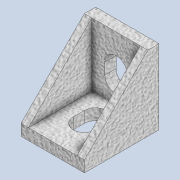
# Autodesk Inventor part: 2020 Extrusion 90deg 2Hole Aluminum Bracket
Saved by Autodesk Inventor 2022 (Build 260153000, 153)
## iProperties
Created: 2021-11-27
Part Number: 2020 Extrusion 90deg 2Hole Aluminum Bracket
Material: Generic
Document SubType Name: Modeling
Designer: Coy
Density: 1 g/cm^3
Appearance: Aluminum Cast
Author: Coy
Autodesk Inventor part; units mm, degrees
ref_plane "YZ Plane" through (0, 0, 0) normal (1, 0, 0) x (0, 1, 0)
ref_plane "XZ Plane" through (0, 0, 0) normal (0, 1, 0) x (-1, 0, 0)
ref_plane "XY Plane" through (0, 0, 0) normal (0, 0, 1) x (1, 0, 0)
sketch "Sketch1" plane through (0, 0, 0) normal (1, 0, 0) x (0, 1, 0)
  line L0 (0, 0) -> (0, 20)
  line L1 (0, 20) -> (3, 20)
  line L2 (3, 20) -> (20, 3)
  line L3 (20, 3) -> (20, 0)
  line L4 (20, 0) -> (0, 0)
  dimension "d0" = 20
  dimension "d1" = 3
  dimension "d2" = 20
  dimension "d3" = 3
  constraints: 10 end point, 2 perpendicular, 1 parallel, 1 vertical
  measures "d0" distance of L0.start L0.end
  measures "d1" distance of L0.end L1.end
  measures "d2" distance of L3.end L0.start
  measures "d3" distance of L2.end L3.end
extrude "Extrusion1" add sketch "Sketch1" along normal blind 2
sketch "Sketch2" plane through (2, 0, 0) normal (1, 0, 0) x (0, 0, -1)
  line L0 (0, 20) -> (-3, 20) projected
  line L1 (-3, 20) -> (-20, 3) projected
  line L2 (-20, 3) -> (-20, 0) projected
  line L3 (-20, 0) -> (0, 0) projected
  line L4 (0, 0) -> (0, 20) projected
  line L5 (-3, 20) -> (-20, 3) projected
  line L6 (-20, 3) -> (-3, 3)
  line L7 (-3, 3) -> (-3, 20)
  constraints: 4 end point, 1 horizontal, 1 perpendicular
extrude "Extrusion2" add sketch "Sketch2" along normal blind 13 contours L4 L3 L2 L6 L7 L0
sketch "Sketch3" plane through (15, 0, 0) normal (1, 0, 0) x (0, 0, -1)
  line L0 (-3, 3) -> (-3, 20) projected
  line L1 (-3, 20) -> (-20, 3) projected
  line L2 (-20, 3) -> (-3, 3) projected
  line L3 (-20, 0) -> (0, 0) projected
  line L4 (0, 0) -> (0, 20) projected
  line L5 (0, 20) -> (-3, 20) projected
  line L6 (-3, 20) -> (-3, 3) projected
  line L7 (-3, 3) -> (-20, 3) projected
  line L8 (-20, 3) -> (-20, 0) projected
extrude "Extrusion3" add sketch "Sketch3" along normal blind 2
sketch "Sketch4" plane through (2, 3, 3) normal (0, 0, 1) x (1, 0, 0)
  line L0 (-2, 17) -> (15, 17) construction
  line L1 (6.5, 17) -> (6.5, 0) construction
  line L2 (0, 0) -> (13, 0) construction
  line L3 (6.5, 11.5) -> (6.5, 2.5) construction
  line L4 (3.5, 8.5) -> (3.5, 5.5)
  line L5 (9.5, 5.5) -> (9.5, 8.5)
  arc A0 (9.5, 8.5) -> (3.5, 8.5) centre (6.5, 8.5) ccw
  arc A1 (3.5, 5.5) -> (9.5, 5.5) centre (6.5, 5.5) ccw
  line L6 (16.0175, -3) -> (16.0175, 17) construction
  line L7 (16.0175, 7) -> (-7.3176, 7) construction
  point P0 (-2, -3)
  point P1 (6.5, 7)
  dimension "d10" = 9
  dimension "d11" = 6
  constraints: 14 end point, 6 point on circle, 5 point on line, 4 midpoint, 4 tangent, 2 centre point, 2 horizontal, 1 parallel, 1 vertical
  measures "d10" distance of L3.start L3.end
  measures "d11" diameter of A1
extrude "Extrusion4" cut sketch "Sketch4" against normal up to next
sketch "Sketch5" plane through (2, 3, 20) normal (0, 1, 0) x (1, 0, 0)
  line L0 (-2, 0) -> (15, 0) construction
  line L1 (6.5, 0) -> (6.5, 20) construction
  line L2 (-2, 20) -> (15, 20) construction
  line L3 (6.5, 5.5) -> (6.5, 14.5) construction
  line L4 (9.5, 8.5) -> (9.5, 11.5)
  line L5 (3.5, 11.5) -> (3.5, 8.5)
  arc A0 (3.5, 8.5) -> (9.5, 8.5) centre (6.5, 8.5) ccw
  arc A1 (9.5, 11.5) -> (3.5, 11.5) centre (6.5, 11.5) ccw
  line L6 (-4.1975, 20) -> (-4.1975, 0) construction
  line L7 (-4.1975, 10) -> (18.4942, 10) construction
  point P0 (6.5, 10)
  dimension "d14" = 9
  dimension "d15" = 6
  constraints: 14 end point, 6 point on circle, 5 point on line, 4 midpoint, 4 tangent, 2 centre point, 2 horizontal, 1 parallel, 1 vertical
  measures "d14" distance of L3.start L3.end
  measures "d15" diameter of A1
extrude "Extrusion5" cut sketch "Sketch5" against normal up to next
body "Solid1"
